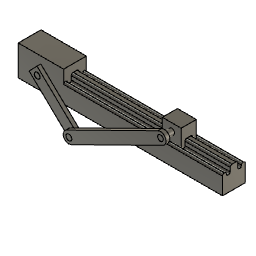
slotted CAM mechanism (Autodesk Fusion 360 design; units mm, degrees)
Autodesk Fusion 360 part; units mm, degrees
sketch "Sketch1" plane through (0, 0, 0) normal (0, 1, 0) x (1, 0, 0) in component "base"
  line L0 (0, 0) -> (120, 0)
  line L1 (120, 0) -> (120, -80)
  line L2 (120, -80) -> (0, -80)
  line L3 (0, -80) -> (0, 0)
  line L4 (120, 0) -> (540, 0)
  line L5 (540, 0) -> (540, -50)
  line L6 (540, -50) -> (120, -50)
  line L7 (120, -50) -> (120, 0)
  dimension "d1" = 120
  dimension "d2" = 80
  dimension "d3" = 420
  dimension "d4" = 50
  constraint horizontal L0
  constraint vertical L1
  constraint horizontal L2
  constraint vertical L3
  constraint coincident L0.start L3.end
  constraint horizontal L4
  constraint vertical L5
  constraint horizontal L6
  constraint vertical L7
  measures "d1" distance of L0.start L0.end
  measures "d2" distance of L0.start L2.end
  measures "d3" distance of L0.end L4.end
  measures "d4" distance of L4 L6
extrude "Extrude1" add sketch "Sketch1" along normal mid plane 60 makes body 1 in component "base"
sketch "Sketch2" plane through (120, 0, 0) normal (1, 0, 0) x (0, 1, 0) in component "base"
  line L0 (-30, 50) -> (30, 50)
  line L1 (30, 50) -> (30, 80)
  line L2 (30, 80) -> (-30, 80)
  line L3 (-30, 80) -> (-30, 50)
  line L4 (-9.7756, 50) -> (10.2244, 50)
  line L5 (10.2244, 50) -> (10.2244, 60)
  line L6 (10.2244, 60) -> (-9.7756, 60)
  line L7 (-9.7756, 60) -> (-9.7756, 50)
  line L8 (-9.7756, 50) -> (-19.7756, 50)
  line L9 (-19.7756, 50) -> (-19.7756, 40)
  line L10 (-19.7756, 40) -> (-9.7756, 40)
  line L11 (-9.7756, 40) -> (-9.7756, 50)
  line L12 (10.2244, 50) -> (20.2244, 50)
  line L13 (20.2244, 50) -> (20.2244, 40)
  line L14 (20.2244, 40) -> (10.2244, 40)
  line L15 (10.2244, 40) -> (10.2244, 50)
  dimension "d7" = 20
  dimension "d8" = 10
  dimension "d9" = 10
  dimension "d10" = 10
  dimension "d11" = 10
  dimension "d12" = 10
  constraint horizontal L4
  constraint vertical L5
  constraint horizontal L6
  constraint vertical L7
  constraint coincident L0 L4.start
  constraint horizontal L8
  constraint vertical L9
  constraint horizontal L10
  constraint vertical L11
  constraint horizontal L12
  constraint vertical L13
  constraint horizontal L14
  constraint vertical L15
  measures "d7" distance of L4.start L4.end
  measures "d8" distance of L4.start L6.end
  measures "d9" distance of L9.end L10.end
  measures "d10" distance of L8.end L9.end
  measures "d11" distance of L13.end L14.end
  measures "d12" distance of L12.end L13.end
extrude "Extrude2" add sketch "Sketch2" along normal blind 420 contours L0 L4 L5 L6 L7 bodies 1 in component "base"
extrude "Extrude3" cut sketch "Sketch2" along normal blind 450 contours L0 L8 L9 L10 L11 | L0 L12 L13 L14 L15 bodies 1 in component "base"
fillet "Fillet1" radius 5 10 edges at (330, -30, 50) (330, -19.7756, 50) (330, -19.7756, 40) (330, -9.7756, 40) (330, -9.7756, 60) (330, 10.2244, 60) (330, 10.2244, 40) (330, 20.2244, 40) (330, 20.2244, 50) (330, 30, 50) on bodies 1 in component "base"
sketch "Sketch3" plane through (0, -30, 0) normal (0, -1, 0) x (1, 0, 0) in component "base"
  line L0 (120, 45) -> (120, 80)
  line L1 (120, 80) -> (0, 80)
  line L2 (0, 80) -> (0, 0)
  line L3 (0, 0) -> (540, 0)
  line L4 (540, 0) -> (540, 45)
  line L5 (540, 45) -> (120, 45)
  circle A0 centre (60, 40) radius 7.5
  dimension "d19" = 15
  dimension "d20" = 60
  dimension "d21" = 40
  measures "d19" diameter of A0
  measures "d20" horizontal distance of L2.end A0.centre
  measures "d21" distance of L3 A0.centre
extrude "Extrude4" add sketch "Sketch3" along normal blind 10 contours A0 bodies 1 in component "base"
sketch "Sketch1 (2)" plane through (0, -30, 0) normal (0, -1, 0) x (1, 0, 0) in component "link 1"
  circle A0 centre (60, 40) radius 7.5
  line L0 (120, 45) -> (120, 80)
  line L1 (120, 80) -> (0, 80)
  line L2 (0, 80) -> (0, 0)
  line L3 (0, 0) -> (540, 0)
  line L4 (540, 0) -> (540, 45)
  line L5 (540, 45) -> (120, 45)
  circle A1 centre (60, 40) radius 7.5
  line L6 (38.7868, 39.9551) -> (60.0449, 18.7868)
  line L7 (60.0449, 18.7868) -> (172.9424, 132.163)
  line L8 (172.9424, 132.163) -> (151.6844, 153.3312)
  line L9 (151.6844, 153.3312) -> (38.7868, 39.9551)
  dimension "d24" = 15
  dimension "d25" = 15
  dimension "d26" = 30
  dimension "d27" = 160
  constraint perpendicular L6 L7
  constraint parallel L6 L8
  constraint parallel L7 L9
  measures "d24" distance of A0.centre L7
  measures "d25" distance of A0.centre L6
  measures "d26" distance of L6.start L6.end
  measures "d27" distance of L6.start L8.end
sketch "Sketch2 (2)" plane through (125.8025, -30, 116.1637) normal (0, -1, 0) x (1, 0, 0) in component "link 1"
  circle A0 centre (25.9386, 15.9426) radius 7.5
  line L0 (47.1399, 15.9993) -> (25.8818, 37.1676)
  dimension "d28" = 15
  dimension "d29" = 15
  measures "d28" diameter of A0
  measures "d29" distance of A0.centre L0
extrude "Extrude1'" add sketch "Sketch1 (2)" along normal blind 10 separate body contours L0 L1 L6 L7 L9 | L0 L1 L7 L8 L9 makes body 2 in component "link 1"
sketch "Sketch3 (2)" plane through (0, -40, 0) normal (0, -1, 0) x (1, 0, 0) in component "link 1"
  circle A0 centre (60, 40) radius 7.5
  line L0 (151.6844, 153.3312) -> (38.7868, 39.9551)
  line L1 (38.7868, 39.9551) -> (60.0449, 18.7868)
  line L2 (60.0449, 18.7868) -> (172.9424, 132.163)
  line L3 (172.9424, 132.163) -> (151.6844, 153.3312)
  circle A1 centre (151.611, 132.0858) radius 7.6058
extrude "Extrude2'" add sketch "Sketch3 (2)" along normal blind 10 contours A1 bodies 2 in component "link 1"
extrude "Extrude3'" cut sketch "Sketch2 (2)" along normal blind 10 bodies 2 in component "link 1"
fillet "Fillet1'" radius 15 2 edges at (172.9424, -35, 132.163) (151.6844, -35, 153.3312) on bodies 2 in component "link 1"
sketch "Sketch1 (3)" plane through (0, -40, 0) normal (0, -1, 0) x (1, 0, 0) in component "link 2"
  arc A0 (162.3583, 121.5339) -> (141.1003, 142.7022) centre (151.7293, 132.1181) ccw
  line L0 (141.1003, 142.7022) -> (38.7868, 39.9551)
  line L1 (38.7868, 39.9551) -> (60.0449, 18.7868)
  line L2 (60.0449, 18.7868) -> (162.3583, 121.5339)
  arc A1 (158.3691, 128.5962) -> (156.9698, 137.4832) centre (151.7411, 132.1063) ccw
  arc A2 (156.9698, 137.4832) -> (158.3691, 128.5962) centre (151.611, 132.0858) ccw
  circle A3 centre (60, 40) radius 7.5
  circle A4 centre (151.611, 132.0858) radius 7.6058
  line L3 (136.611, 147.0858) -> (436.611, 147.0858)
  line L4 (436.611, 147.0858) -> (436.611, 117.0858)
  line L5 (436.611, 117.0858) -> (136.611, 117.0858)
  line L6 (136.611, 117.0858) -> (136.611, 147.0858)
  dimension "d38" = 30
  dimension "d39" = 300
  dimension "d40" = 15
  dimension "d41" = 15
  constraint horizontal L3
  constraint vertical L4
  constraint horizontal L5
  constraint vertical L6
  measures "d38" distance of L3.start L5.end
  measures "d39" distance of L3.start L3.end
  measures "d40" distance of A2.centre L5
  measures "d41" distance of A2.centre L6
extrude "Extrude1''" add sketch "Sketch1 (3)" along normal blind 10 separate body contours A0 L0 L2 L3 L5 L6 | A0 L2 L3 L4 L5 | A0 L0 L3 L6 makes body 3 in component "link 2"
fillet "Fillet1''" radius 15 3 edges at (136.611, -45, 117.0858) (436.611, -45, 147.0858) (436.611, -45, 117.0858) on bodies 3 in component "link 2"
fillet "Fillet2" radius 15 1 edges at (136.611, -45, 147.0858) on bodies 3 in component "link 2"
hole "Hole1" at (421.611, -50, 132.0858) direction (0, 1, 0) diameter 15 end through all bodies 3 in component "link 2"
sketch "Sketch1 (4)" plane through (540, 0, 0) normal (1, 0, 0) x (0, 1, 0) in component "slider"
  arc A0 (30, 45.005) -> (25.2244, 50) centre (25, 45.005) ccw
  arc A1 (25.2244, 50) -> (20.2244, 45) centre (25.2244, 45) ccw
  arc A2 (10.2244, 45) -> (20.2244, 45) centre (15.2244, 45) ccw
  line L0 (10.2244, 45) -> (10.2244, 55)
  arc A3 (10.2244, 55) -> (5.2244, 60) centre (5.2244, 55) ccw
  line L1 (5.2244, 60) -> (-4.7756, 60)
  arc A4 (-4.7756, 60) -> (-9.7756, 55) centre (-4.7756, 55) ccw
  line L2 (-9.7756, 55) -> (-9.7756, 45)
  arc A5 (-19.7756, 45) -> (-9.7756, 45) centre (-14.7756, 45) ccw
  arc A6 (-19.7756, 45) -> (-24.7756, 50) centre (-24.7756, 45) ccw
  line L3 (-24.7756, 50) -> (-25, 50)
  arc A7 (-25, 50) -> (-30, 45) centre (-25, 45) ccw
  line L4 (-30, 45) -> (-30, 0)
  line L5 (-30, 0) -> (30, 0)
  line L6 (30, 0) -> (30, 45.005)
  line L7 (-19.7756, 40) -> (20.2244, 40)
  line L8 (20.2244, 40) -> (20.2244, 90)
  line L9 (20.2244, 90) -> (-19.7756, 90)
  line L10 (-19.7756, 90) -> (-19.7756, 40)
  dimension "d51" = 50
  dimension "d52" = 40
  constraint horizontal L7
  constraint vertical L8
  constraint horizontal L9
  constraint vertical L10
  measures "d51" distance of L7.start L9.end
  measures "d52" distance of L7.start L7.end
extrude "Extrude1'''" add sketch "Sketch1 (4)" against normal blind 50 separate body contours A2 L0 A3 L1 A4 L2 A5 L8 L9 L10 makes body 4 in component "slider"
sketch "Sketch1 (5)" plane through (0, -19.7756, 0) normal (0, -1, 0) x (1, 0, 0)
  line L0 (540, 45) -> (540, 90)
  line L1 (540, 90) -> (490, 90)
  line L2 (490, 90) -> (490, 45)
  line L3 (490, 45) -> (540, 45)
  circle A0 centre (515, 70) radius 7.5
  dimension "d55" = 15
  measures "d55" diameter of A0
extrude "Extrude2''" add sketch "Sketch1 (5)" along normal blind 30 contours A0 bodies 4 in component "slider"
component "base" placed x (1, 0, 0) y (0, 1, 0) z (0, 0, 1) at (0, 0, 0)
component "link 2" placed x (0.983767, 0, -0.179449) y (0, 1, 0) z (0.179449, 0, 0.983767) at (-9.8267, 0.2244, 15.7158)
component "slider" placed x (1, 0, 0) y (0, 1, 0) z (0, 0, 1) at (-86.3569, 0, 0)
component "link 1" placed x (0.990531, 0, -0.137293) y (0, 1, 0) z (0.137293, 0, 0.990531) at (-5.2839, 0.2244, 8.4312) in component "base"
